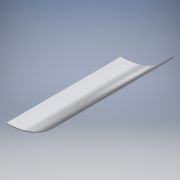
# Autodesk Inventor part: Part4
Saved by Autodesk Inventor 2016 (Build 200138000, 138)
## iProperties
Created: 2016-09-04
Part Number: Part4
Material: Aluminum 6061
Document SubType Name: Modeling
Designer: gus
Density: 2.7 g/cm^3
Appearance: Aluminum - Flat
Author: gus
Autodesk Inventor part; units mm, degrees
ref_plane "YZ Plane" through (0, 0, 0) normal (1, 0, 0) x (0, 1, 0)
ref_plane "XZ Plane" through (0, 0, 0) normal (0, 1, 0) x (-1, 0, 0)
ref_plane "XY Plane" through (0, 0, 0) normal (0, 0, 1) x (1, 0, 0)
sketch "Sketch1" plane through (0, 0, 0) normal (0, 0, 1) x (1, 0, 0)
  arc A0 (0, 0) -> (177.8, 88.9) centre (0, 222.25) ccw
  line L0 (0, 0) -> (177.8, 0) construction
  arc A1 (0, 3.175) -> (177.8, 94.2617) centre (0, 222.25) ccw
  line L1 (0, 3.175) -> (0, 0)
  line L2 (177.8, 88.9) -> (177.8, 94.2617)
  dimension "d0" = 222.25
  dimension "d7" = 3.175
  dimension "d9" = 3.175
  dimension "d12" = 177.8
  dimension "d13" = 177.8
  constraints: 6 end point, 4 point on circle, 2 centre point, 1 concentric, 1 horizontal, 1 tangent, 1 vertical
  measures "d0" radius of A0
  measures "d7" radial gap between concentric circles of A0 A1
  measures "d9" distance of L1.start L0.start
  measures "d12" distance of L0.start L0.end
  measures "d13" horizontal distance of L0.start L2.end
extrude "Extrusion1" add sketch "Sketch1" against normal blind 539.75
sketch "Sketch2" plane through (0, 0, 0) normal (0, 0, 1) x (1, 0, 0)
  arc A0 (0, 0) -> (177.8, 88.9) centre (0, 222.25) ccw projected
  line L0 (177.8, 88.9) -> (177.8, 232.5642)
  line L1 (177.8, 232.5642) -> (0, 222.25)
  line L2 (0, 222.25) -> (0, 0)
  dimension "d14" = 93.32
  dimension "d15" = 0
  constraints: 6 end point, 2 vertical
  measures "d14" angle of L1 L2
  measures "d15" distance from line of L1 A0.centre
extrude "Extrusion2" add sketch "Sketch2" along normal blind 3.175
ref_plane "Work Plane1" through (0, 0, -269.875) normal (0, 0, -1) x (-1, 0, 0)
mirror "Mirror1" about plane through (0, 0, -269.875) normal (0, 0, -1) of "Extrusion2"
sketch "Sketch3" plane through (177.8, 94.2617, 0) normal (1, 0, 0) x (0, 0, -1)
  line L0 (542.925, -5.3617) -> (-3.175, -5.3617) projected
  line L1 (-3.175, 138.3025) -> (95.25, 138.3025)
  line L2 (95.25, 138.3025) -> (95.25, -5.3617)
  line L3 (95.25, -5.3617) -> (-3.175, -5.3617)
  line L4 (-3.175, -5.3617) -> (-3.175, 138.3025)
  line L5 (0, 138.3025) -> (-3.175, 138.3025) projected
  line L6 (-3.175, -5.3617) -> (-3.175, 138.3025) projected
  line L7 (542.925, -5.3617) -> (444.5, -5.3617)
  line L8 (444.5, -5.3617) -> (444.5, 138.3025)
  line L9 (444.5, 138.3025) -> (542.925, 138.3025)
  line L10 (542.925, 138.3025) -> (542.925, -5.3617)
  line L11 (539.75, 138.3025) -> (542.925, 138.3025) projected
  point P0 (0, -94.2617)
  dimension "d19" = 98.425
  dimension "d20" = 98.425
  constraints: 16 end point, 4 parallel, 3 collinear, 2 horizontal, 2 perpendicular, 1 point on line
  measures "d19" distance of L1.start L1.end
  measures "d20" distance of L8.end L9.end
extrude "Extrusion3" add sketch "Sketch3" along normal blind 3.175
body "Solid1"
